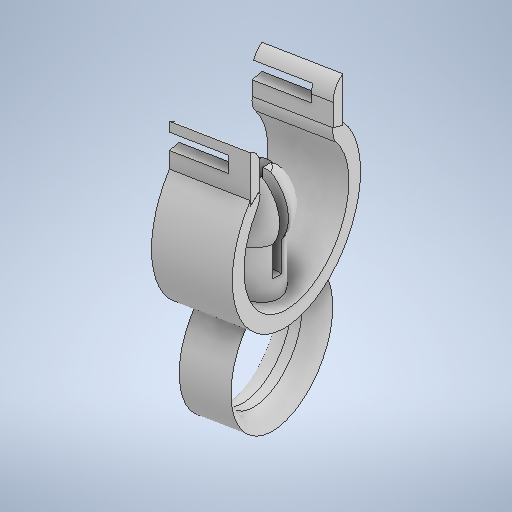
# Autodesk Inventor part: Clip2
Saved by Autodesk Inventor 2025 (Build 290162010, 162A)
## iProperties
Created: 2026-02-19
Part Number: Clip2
Material: Generic
Document SubType Name: Modeling
Designer: 925699
Density: 1 g/cm^3
Appearance: Default
Author: 925699
Autodesk Inventor part; units mm, degrees
ref_plane "YZ Plane" through (0, 0, 0) normal (1, 0, 0) x (0, 1, 0)
sketch "Sketch1" plane through (0, 0, 0) normal (0, 0, 1) x (1, 0, 0)
  line L0 (0, 0) -> (4.064, 0)
  line L1 (4.064, 0) -> (4.064, 8.6967)
  line L2 (2.2474, 17.8837) -> (0, 17.8837)
  line L3 (0, 0) -> (0, 17.8837)
  arc A0 (4.064, 8.6967) -> (2.2474, 17.8837) centre (-1.2362, 12.4217) ccw
  dimension "d0" = 4.064
  constraints: 8 end point, 2 horizontal, 2 point on circle, 1 centre point, 1 perpendicular, 1 vertical
  measures "d0" distance of L0.start L0.end
revolve "Revolution1" add sketch "Sketch1" angle 360 about axis through (0, 0, 0) along (0, 1, 0)
sketch "Sketch2" plane through (0, 17.8837, 0) normal (0, 1, 0) x (1, 0, 0)
  line L0 (-6.4086, -0.7741) -> (9.1253, -0.7741)
  line L1 (9.1253, -0.7741) -> (9.1253, 0.7499)
  line L2 (9.1253, 0.7499) -> (-6.4086, 0.7499)
  line L3 (-6.4086, 0.7499) -> (-6.4086, -0.7741)
  line L4 (0.7741, -6.4086) -> (0.7741, 9.1253)
  line L5 (0.7741, 9.1253) -> (-0.7499, 9.1253)
  line L6 (-0.7499, 9.1253) -> (-0.7499, -6.4086)
  line L7 (-0.7499, -6.4086) -> (0.7741, -6.4086)
  point P0 (0, 0)
  point P1 (-0.7499, -0.7741)
  point P2 (0.7741, -0.7741)
  point P3 (0.7741, 0.7499)
  point P4 (-0.7499, 0.7499)
  dimension "d3" = 1.524
  dimension "d6" = 90
  constraints: 16 end point, 2 parallel, 1 horizontal, 1 perpendicular, 9 other
  measures "d3" distance of L1.end L0.end
extrude "Extrusion1" cut sketch "Sketch2" against normal blind 14.2875
ref_plane "Work Plane1" through (-3.9896, 4.3483, 0.7741) normal (-0.9816919, 0, 0.1904757) x (0, -1, 0)
sketch "Sketch3" plane through (-3.9896, 4.3483, 0.7741) normal (-0.9816919, 0, 0.1904757) x (0, -1, 0)
  arc A0 (-16.337, -6.8791) -> (-16.337, 6.8791) centre (-7.2089, 0) ccw
  arc A1 (-18.3655, -8.4078) -> (-18.3655, 8.4078) centre (-7.2089, 0) ccw
  line L0 (-13.5354, -0.5887) -> (0.7521, -0.5887) projected
  line L1 (-13.5354, 0.6171) -> (0.7521, 0.6171) projected
  line L2 (-7.2089, 0) -> (-7.9901, -0.5887)
  line L3 (-16.337, -6.8791) -> (-18.3655, -8.4078)
  line L4 (-7.2089, 0) -> (-8.0277, 0.6171)
  line L5 (-16.337, 6.8791) -> (-18.3655, 8.4078)
  constraints: 8 end point, 4 point on circle, 2 centre point, 2 coincident, 2 point on line
extrude "Extrusion2" add sketch "Sketch3" along normal blind 1.5875 and the other way blind 10.3124
fillet "Fillet1" radius 3.175 2 edges at (-1.0173, 20.6854, -6.81) (1.6033, 20.6854, 6.6963)
ref_plane "Work Plane2" through (0.293, 4.3483, -0.0568) normal (0.9816919, 0, -0.1904757) x (-0.1904757, 0, -0.9816919)
sketch "Sketch4" plane through (0.293, 4.3483, -0.0568) normal (0.9816919, 0, -0.1904757) x (-0.1904757, 0, -0.9816919)
  circle A0 centre (0, -12.1867) radius 8.89
  arc A1 (-8.4078, 18.3655) -> (8.4078, 18.3655) centre (0, 7.2089) ccw projected
  arc A2 (-7.848, -4.3483) -> (7.848, -4.3483) centre (0, -12.1867) ccw
  point P0 (0, -4.3483)
  point P1 (5.8384, -5.4826)
  point P2 (-5.8384, -5.4826)
  dimension "d17" = 17.78
  constraints: 4 point on circle, 2 centre point, 1 concentric
  measures "d17" diameter of A0
extrude "Extrusion3" add sketch "Sketch4" along normal mid plane 7.62 contours A0 A1 A2
fillet "Fillet2" radius 3.175 2 edges at (-3.4473, -16.7283, 0.6689) (4.0332, -16.7283, -0.7826)
sketch "Sketch5" plane through (-5.548, 4.3483, 1.0765) normal (-0.9816919, 0, 0.1904757) x (0.1904757, 0, 0.9816919)
  arc A0 (-8.6921, 14.6313) -> (-8.4078, 18.3655) centre (-11.1066, 16.6931) ccw projected
  line L0 (-7.9735, 17.2071) -> (-7.9735, 24.0368)
  line L1 (-7.9735, 24.0368) -> (-10.116, 24.0368)
  line L2 (-10.116, 24.0368) -> (-10.116, 16.3667)
  arc A1 (8.4078, 18.3655) -> (8.6921, 14.6313) centre (11.1066, 16.6931) ccw projected
  line L3 (7.9735, 17.2071) -> (7.9735, 24.0368)
  line L4 (7.9735, 24.0368) -> (10.0556, 24.0368)
  line L5 (10.0556, 24.0368) -> (10.0556, 16.0648)
  line L6 (-10.116, 16.3667) -> (-7.9735, 17.2071)
  line L7 (7.9735, 17.2071) -> (10.0556, 16.0648)
  point P0 (0, -4.3483)
  constraints: 16 end point, 4 perpendicular, 2 point on circle, 2 vertical
extrude "Extrusion4" add sketch "Sketch5" against normal blind 11.9126
sketch "Sketch6" plane through (-5.548, 4.3483, 1.0765) normal (-0.9816919, 0, 0.1904757) x (0.1904757, 0, 0.9816919)
  line L0 (11.5164, 22.4175) -> (-13.6635, 22.4175)
  line L1 (-13.6635, 22.4175) -> (-13.6635, 19.6848)
  line L2 (-13.6635, 19.6848) -> (11.5164, 19.6848)
  line L3 (11.5164, 19.6848) -> (11.5164, 22.4175)
  point P0 (0, -4.3483)
  constraints: 8 end point, 2 parallel, 1 horizontal, 1 perpendicular
extrude "Extrusion5" cut sketch "Sketch6" against normal blind 8.7376
fillet "Fillet3" radius 3.175 2 edges at (1.818, 28.3851, 7.7695) (-1.2195, 28.3851, -7.8856)
body "Solid1"
